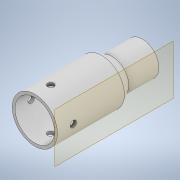
# Autodesk Inventor part: fuel
Saved by Autodesk Inventor 2021 (Build 250183000, 183)
## iProperties
Created: 2023-07-01
Part Number: fuel
Material: Generic
Document SubType Name: Modeling
Designer: harsh
Density: 1 g/cm^3
Appearance: Default
Author: harsh
Autodesk Inventor part; units mm, degrees
ref_plane "XZ Plane" through (0, 0, 0) normal (0, 1, 0) x (-1, 0, 0)
ref_plane "XY Plane" through (0, 0, 0) normal (0, 0, 1) x (1, 0, 0)
sketch "Sketch1" plane through (0, 0, 0) normal (1, 0, 0) x (0, 1, 0)
  line L0 (6.2, 1.0944) -> (6.2, -19.7056)
  line L1 (4.3, -32.6965) -> (4.3, -22.9965)
  line L2 (6.2, -19.7056) -> (4.3, -22.9965)
  line L3 (7.1, -19.9467) -> (7.1, 1.0944)
  line L4 (5.2, -32.6965) -> (5.2, -23.2376)
  line L5 (5.2, -23.2376) -> (7.1, -19.9467)
  line L6 (6.2, 1.0944) -> (7.1, 1.0944)
  line L7 (4.3, -32.6965) -> (5.2, -32.6965)
  line L8 (0, 0) -> (0, -7.1245) construction
  dimension "d5" = 6.2
  dimension "d6" = 4.3
  dimension "d7" = 0.9
  dimension "d8" = 0.9
  dimension "d9" = 0.9
  dimension "d10" = 20.8
  dimension "d11" = 9.7
  dimension "d12" = 150
  constraints: 18 end point, 1 horizontal, 1 perpendicular, 1 vertical
  measures "d5" distance between parallel lines of L0 L8
  measures "d6" distance between parallel lines of L1 L8
  measures "d7" distance between parallel lines of L3 L0
  measures "d8" distance between parallel lines of L5 L2
  measures "d9" distance between parallel lines of L4 L1
  measures "d10" distance of L0.start L0.end
  measures "d11" distance of L1.start L1.end
  measures "d12" angle of L2 L0
revolve "Revolution1" add sketch "Sketch1" angle 360 about axis through (0, 0, 0) along (0, 0, -1)
ref_plane "Work Plane1" through (8, 0, 0) normal (1, 0, 0) x (0, 1, 0)
sketch "Sketch2" plane through (8, 0, 0) normal (1, 0, 0) x (0, 1, 0)
  line L0 (0, 1.0944) -> (0, -3.9056) construction
  circle A0 centre (0, -3.9056) radius 1
  point P0 (0, 0)
  dimension "d15" = 5
  dimension "d16" = 2
  constraints: 2 end point, 1 centre point, 1 coincident, 1 vertical
  measures "d15" distance of L0.start L0.end
  measures "d16" diameter of A0
extrude "Extrusion1" cut sketch "Sketch2" against normal blind 10
pattern_circular "Circular Pattern1" count 4 over 360 about axis through (0, 0, -21.351) along (0, 0, -1) of "Extrusion1"
body "Solid1"
